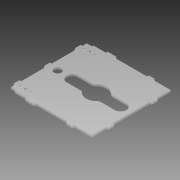
# Autodesk Inventor part: plastic_part_04
Saved by Autodesk Inventor 2013 (Build 170138000, 138)
## iProperties
Shininess: 20.0
Created: 2013-02-12
Part Number: plastic_part_04
Document SubType Name: Modeling
Designer: Noa Izumi
Material: Default
Density: 1 g/cm^3
Density: 0.0
Volumn: 0.0
Area: 0.0
PropertySet Name: Model Information
Control State: 0
Master: False
Checked Out: False
Author: Noa Izumi
Autodesk Inventor part; units mm, degrees
ref_plane "YZ Plane" through (0, 0, 0) normal (1, 0, 0) x (0, 1, 0)
ref_plane "XZ Plane" through (0, 0, 0) normal (0, 1, 0) x (-1, 0, 0)
ref_plane "XY Plane" through (0, 0, 0) normal (0, 0, 1) x (1, 0, 0)
sketch "Sketch1" plane through (0, 0, 0) normal (0, 0, 1) x (1, 0, 0)
  line L0 (0, 0) -> (140, 0)
  line L1 (140, 0) -> (140, 134)
  line L2 (140, 134) -> (0, 134)
  line L3 (0, 134) -> (0, 0)
  line L4 (30, 137) -> (45, 137)
  line L5 (45, 137) -> (45, -3)
  line L6 (45, -3) -> (30, -3)
  line L7 (30, -3) -> (30, 137)
  line L8 (100, 137) -> (110, 137)
  line L9 (110, 137) -> (110, -3)
  line L10 (110, -3) -> (100, -3)
  line L11 (100, -3) -> (100, 137)
  line L12 (-3, 124) -> (0, 124)
  line L13 (0, 124) -> (0, 114)
  line L14 (0, 114) -> (-3, 114)
  line L15 (-3, 114) -> (-3, 124)
  line L16 (-3, 20) -> (0, 20)
  line L17 (0, 20) -> (0, 10)
  line L18 (0, 10) -> (-3, 10)
  line L19 (-3, 10) -> (-3, 20)
  line L20 (-3, 72) -> (0, 72)
  line L21 (0, 72) -> (0, 62)
  line L22 (0, 62) -> (-3, 62)
  line L23 (-3, 62) -> (-3, 72)
  line L24 (140, 109) -> (143, 109)
  line L25 (143, 109) -> (143, 99)
  line L26 (143, 99) -> (140, 99)
  line L27 (140, 99) -> (140, 109)
  line L28 (140, 35) -> (143, 35)
  line L29 (143, 35) -> (143, 25)
  line L30 (143, 25) -> (140, 25)
  line L31 (140, 25) -> (140, 35)
  dimension "d0" = 140
  dimension "d1" = 134
  dimension "d2" = 140
  dimension "d3" = 3
  dimension "d4" = 15
  dimension "d5" = 10
  dimension "d6" = 140
  dimension "d7" = 3
  dimension "d8" = 30
  dimension "d9" = 30
  dimension "d10" = 10
  dimension "d11" = 3
  dimension "d13" = 10
  dimension "d14" = 3
  dimension "d16" = 10
  dimension "d17" = 10
  dimension "d74" = 10
  dimension "d75" = 42
  dimension "d76" = 3
  dimension "d77" = 10
  dimension "d78" = 3
  dimension "d79" = 25
  dimension "d80" = 10
  dimension "d81" = 25
  dimension "d82" = 3
  constraints: 64 end point, 16 parallel, 8 horizontal, 8 perpendicular, 2 point on line
  measures "d0" distance of L0.start L0.end
  measures "d1" distance of L2.end L0.start
  measures "d2" distance of L6.end L4.start
  measures "d3" distance between parallel lines of L6 L0
  measures "d4" distance of L5.end L6.end
  measures "d5" distance of L9.end L10.end
  measures "d6" distance of L8.end L9.end
  measures "d7" distance between parallel lines of L10 L0
  measures "d8" distance between parallel lines of L7 L3
  measures "d9" distance between parallel lines of L1 L9
  measures "d10" distance of L14.end L12.start
  measures "d11" distance of L12.start L12.end
  measures "d13" distance of L18.end L16.start
  measures "d14" distance between parallel lines of L3 L19
  measures "d16" distance between parallel lines of L2 L12
  measures "d17" distance between parallel lines of L0 L18
  measures "d74" distance of L22.end L20.start
  measures "d75" distance between parallel lines of L20 L14
  measures "d76" distance of L21.end L22.end
  measures "d77" distance of L24.end L25.end
  measures "d78" distance of L24.start L24.end
  measures "d79" distance from line of L24.end L2
  measures "d80" distance of L28.end L29.end
  measures "d81" distance from line of L29.end L0
  measures "d82" distance of L28.start L28.end
extrude "Extrusion1" add sketch "Sketch1" along normal blind 3
sketch "Sketch2" plane through (0, 0, 3) normal (0, 0, 1) x (1, 0, 0)
  line L0 (40, 77) -> (122, 77)
  line L1 (132, 67) -> (132, 67)
  line L2 (122, 57) -> (40, 57)
  line L3 (30, 67) -> (30, 67)
  arc A0 (40, 77) -> (30, 67) centre (40, 67) ccw
  arc A1 (30, 67) -> (40, 57) centre (40, 67) ccw
  arc A2 (122, 57) -> (132, 67) centre (122, 67) ccw
  arc A3 (132, 67) -> (122, 77) centre (122, 67) ccw
  line L4 (140, 114) -> (140, 20) projected
  line L5 (45, 134) -> (100, 134) projected
  circle A4 centre (81, 67) radius 17.5
  point P0 (30, 77)
  point P1 (132, 77)
  point P2 (30, 57)
  dimension "d20" = 20
  dimension "d21" = 102
  dimension "d23" = 10
  dimension "d52" = 8
  dimension "d71" = 57
  dimension "d83" = 35
  dimension "d84" = 51
  constraints: 8 end point, 8 point on circle, 8 tangent, 6 point on line, 5 centre point, 3 equal radius, 2 parallel, 1 horizontal, 1 perpendicular
  measures "d20" distance of point (30, 57) point (30, 77)
  measures "d21" distance of point (30, 77) point (132, 77)
  measures "d23" radius of A0
  measures "d52" distance from line of L4 L1.end
  measures "d71" distance between parallel lines of L0 L5
  measures "d83" diameter of A4
  measures "d84" distance of A4.centre L3.end
extrude "Extrusion2" cut sketch "Sketch2" against normal through all
sketch "Sketch3" plane through (0, 0, 3) normal (0, 0, 1) x (1, 0, 0)
  line L0 (0, 20) -> (0, 114) projected
  line L1 (0, 0) -> (0, 10) projected
  line L2 (30, 0) -> (0, 0) projected
  line L3 (0, 134) -> (30, 134) projected
  point P0 (15, 12)
  point P1 (15, 122)
  dimension "d26" = 15
  dimension "d27" = 12
  dimension "d28" = 15
  dimension "d48" = 12
  measures "d26" distance from line of point (15, 12) L1
  measures "d27" distance from line of point (15, 12) L2
  measures "d28" distance from line of L0 point (15, 122)
  measures "d48" distance from line of point (15, 122) L3
hole "Hole1" at (15, 12, 3) at (15, 122, 3) direction (0, 0, -1) diameter 4 end through all
sketch "Sketch4" plane through (0, 0, 3) normal (0, 0, 1) x (1, 0, 0)
  circle A0 centre (15, 12) radius 2 projected
  circle A1 centre (15, 122) radius 2 projected
  point P0 (24, 122)
  point P1 (6, 122)
  point P2 (24, 12)
  point P3 (6, 12)
  dimension "d37" = 9
  dimension "d38" = 9
  dimension "d39" = 9
  dimension "d40" = 9
  dimension "d49" = 0
  dimension "d50" = 0
  measures "d37" distance of A1.centre point (6, 122)
  measures "d38" distance of point (24, 122) A1.centre
  measures "d39" distance of A0.centre point (6, 12)
  measures "d40" distance of point (24, 12) A0.centre
  measures "d49" vertical distance of A0.centre point (6, 12)
  measures "d50" vertical distance of A1.centre point (6, 122)
hole "Hole2" at (24, 122, 3) at (6, 122, 3) at (24, 12, 3) at (6, 12, 3) direction (0, 0, -1) diameter 3 end through all
sketch "Sketch5" plane through (0, 0, 3) normal (0, 0, 1) x (1, 0, 0)
  point P0 (15, 67)
hole "Hole3" at (15, 67, 3) direction (0, 0, -1) diameter 13 end through all
fillet "圓角1" radius 5 4 edges at (66.6386, 77, 1.5) (95.3614, 77, 1.5) (95.3614, 57, 1.5) (66.6386, 57, 1.5)
sketch "草圖7" plane through (0, 0, 3) normal (0, 0, 1) x (1, 0, 0)
  line L0 (0, 134) -> (9.175, 134)
  line L1 (9.175, 134) -> (9.175, 132.75)
  line L2 (7.925, 131.5) -> (0, 131.5)
  line L3 (0, 131.5) -> (0, 134)
  arc A0 (7.925, 131.5) -> (9.175, 132.75) centre (7.925, 132.75) ccw
  line L4 (0, 0) -> (9.175, 0)
  line L5 (9.175, 0) -> (9.175, 1.25)
  line L6 (7.925, 2.5) -> (0, 2.5)
  line L7 (0, 2.5) -> (0, 0)
  arc A1 (9.175, 1.25) -> (7.925, 2.5) centre (7.925, 1.25) ccw
  point P0 (9.175, 131.5)
  point P1 (9.175, 2.5)
  dimension "d86" = 9.175
  dimension "d88" = 2.5
  dimension "d89" = 1.25
  dimension "d90" = 9.175
  dimension "d91" = 2.5
  dimension "d92" = 1.25
  constraints: 16 end point, 4 parallel, 4 point on circle, 4 point on line, 4 tangent, 2 centre point, 2 horizontal, 2 perpendicular
  measures "d86" distance of point (9.175, 131.5) L2.end
  measures "d88" distance of L0.end point (9.175, 131.5)
  measures "d89" radius of A0
  measures "d90" distance of point (9.175, 2.5) L6.end
  measures "d91" distance of L4.end point (9.175, 2.5)
  measures "d92" radius of A1
extrude "擠出3" cut sketch "草圖7" against normal through all
equation "\"d93\" = d88"
